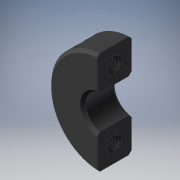
# Autodesk Inventor part: PSCSPJ6-6p
Saved by Autodesk Inventor 2019 (Build 230136000, 136)
## iProperties
Created: 2023-10-07
Part Number: PSCSPJ6-6p
Material: Generic
Catalog Web Link: www.cadenas.de
Description: SCSPJ, PSCSPJ, SSCSPJ, SCNPAJ, SCNPAWJ_p-Set Collars - Separate - Standard Compact Type
Vendor: MISUMI
Document SubType Name: Modeling
Designer: psAdmin
Manufacturer: MISUMI
Mass: 0.589904 g
Surface Area: 5.41828 cm^2
Volume: 0.589904 cm^3
Density: 1 g/cm^3
Appearance: PSOLRGB-191-191-191
Category: PARTsolutions
Company: MISUMI
Title: PSCSPJ6-6p
Author: Cadenas PARTsolutions
Comments: Set Collars - Separate - Standard Compact Type
PSOL_IDENT_0: {$CADENAS_DATA/23d-libs/misumi/metric/03_set_collars/scspj/scspj_p.prj},201 {VTYP=3D},{NB=PSCSPJ6-6p
PSOL_IDENT_1: },{LINA=PSCSPJ6-6p},{NN=SCSPJ, PSCSPJ, SSCSPJ, SCNPAJ, SCNPAWJ_p},{DATE=18.06.2021 05:26:46},{GEOMDA
PSOL_IDENT_2: TE=08.06.2021 05:25:09},{VERSION=},{LINEID=280},{WBVAR=MAT,ST},{WBNUMERIC=}  {NB=PSCSPJ6-6p},{LINA=P
PSOL_IDENT_3: SCSPJ6-6p},{KT=DUMMY},{PN=PSCSPJ6-6},{TYPE=PSCSPJ},{MAT=1},{MATALG='1','1045 Carbon Steel','2','SUS3
PSOL_IDENT_4: 04 Equivalent','3','2017 Aluminum Alloy'},{ST=2},{STALG='1','Black Oxide','2','Electroless Nickel Pl
PSOL_IDENT_5: ating'},{AC=Hexagon Socket Head Cap Screw 1 Pc. (SUS)},{D=6},{B=6},{D1=18.0},{M=M2.6},{M1=2.6},{DD=2
PSOL_IDENT_6: .9},{R=2.45},{W=1.0},{X=6.0},{Y=3.0},{C=0.5},{L=6},{MATA=  'S45C','S45C(1045 Steel)(1.1191_C45E (Ck4
PSOL_IDENT_7: 5))','SUS304','SUS304(304 Stainless Steel)(1.4301_X5CrNi18-10)'    },{COLOR=0.75,0.75,0.75,0.00}
NB: PSCSPJ6-6p
NN: SCSPJ, PSCSPJ, SSCSPJ, SCNPAJ, SCNPAWJ_p
NT: Set Collars - Separate - Standard Compact Type
NBSYN: $PN.p
LINA: PSCSPJ6-6p
CATALOG: Misumi
PN: PSCSPJ6-6
MAT: 1045 Carbon Steel
ST: Electroless Nickel Plating
AC: Hexagon Socket Head Cap Screw 1 Pc. (SUS)
D: 6
B: 6
D1: 18
M: M2.6
DD: 2.9
R: 2.45
W: 1
X: 6
Y: 3
C: 0.5
SUPPLIER: MISUMI
ARTICLENO: PSCSPJ6-6p
BOMINFO: PSCSPJ6-6p
CREATOR: CADENAS GmbH
Autodesk Inventor part; units mm, degrees
sketch "Sketch_1" plane through (0, 0, 0) normal (1, 0, 0) x (0, 1, 0)
  line L0 (0, -3) -> (0, 3)
  line L1 (8.5, 3) -> (3.5, 3)
  line L2 (3.5, 3) -> (3, 2.5)
  line L3 (3, 2.5) -> (3, -2.5)
  line L4 (3, -2.5) -> (3.5, -3)
  line L5 (3.5, -3) -> (8.5, -3)
  line L6 (8.5, -3) -> (9, -2.5)
  line L7 (9, -2.5) -> (9, 2.5)
  line L8 (9, 2.5) -> (8.5, 3)
  constraints: 18 end point
revolve "Revolution1" add sketch "Sketch_1" angle 180 about axis through (0, 0, -3) along (0, 0, 1)
sketch "Sketch_2" plane through (0, 0, 0) normal (0, 0, 1) x (1, 0, 0)
  line L0 (-0.5, -10) -> (0.5, -10)
  line L1 (0.5, -10) -> (0.5, 10)
  line L2 (0.5, 10) -> (-0.5, 10)
  line L3 (-0.5, 10) -> (-0.5, -10)
  constraints: 8 end point
extrude "Extrusion1" cut sketch "Sketch_2" along normal mid plane 6
sketch "Sketch3" plane through (-0.5, -8.4853, -3) normal (1, 0, 0) x (0, 0, -1)
  point P0 (-3, 2.4853)
hole "Hole1" at (-0.5, -6, 0) direction (-1, 0, 0) diameter 2.1129 depth 9 countersink diameter 2.6 countersink angle 90 thread size "M2.6x0.45" class "6H" standard "ISO Metric profile"
sketch "Sketch4" plane through (-0.5, 3.4641, 3) normal (1, 0, 0) x (0, 0, -1)
  point P0 (3, 2.5359)
hole "Hole2" at (-0.5, 6, 0) direction (-1, 0, 0) diameter 2.1129 depth 9 countersink diameter 2.6 countersink angle 90 thread size "M2.6x0.45" class "6H" standard "ISO Metric profile"
ref_plane "2_1_XY" through (0, 0, 0) normal (1, 0, 0) x (0, 0, -1)
ref_plane "2_1_YZ" through (0, 0, 0) normal (0, 0, -1) x (0, 1, 0)
ref_plane "2_1_ZX" through (0, 0, 0) normal (0, 1, 0) x (1, 0, 0)
body "Solid1"
